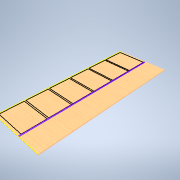
# Autodesk Inventor part: Onderkant1
Saved by Autodesk Inventor 2021 (Build 250183000, 183)
## iProperties
Created: 2021-03-18
Part Number: Onderkant1
Material: Wood (Cherry)
Document SubType Name: Modeling
Designer: ZiweZhang
Density: 0.63 g/cm^3
Appearance: Cherry - Natural Low Gloss
Author: ZiweZhang
Autodesk Inventor part; units mm, degrees
ref_plane "YZ Plane" through (0, 0, 0) normal (1, 0, 0) x (0, 1, 0)
ref_plane "XZ Plane" through (0, 0, 0) normal (0, 1, 0) x (-1, 0, 0)
ref_plane "XY Plane" through (0, 0, 0) normal (0, 0, 1) x (1, 0, 0)
sketch "Sketch1" plane through (0, 0, 0) normal (0, 1, 0) x (-1, 0, 0)
  line L0 (181, 491) -> (-181, 491)
  line L1 (-181, 491) -> (-181, -491)
  line L2 (-181, -491) -> (181, -491)
  line L3 (181, -491) -> (181, 491)
  line L4 (181, 491) -> (-181, -491) construction
  line L5 (-181, 491) -> (181, -491) construction
  point P0 (0, 0)
  dimension "d0" = 362
  dimension "d1" = 982
  constraints: 12 end point, 2 midpoint, 2 parallel, 1 horizontal, 1 perpendicular
  measures "d0" distance of L2.end L1.end
  measures "d1" distance of L1.end L0.end
extrude "Extrusion1" add sketch "Sketch1" along normal blind 6
sketch "Sketch2" plane through (0, 6, 0) normal (0, 1, 0) x (1, 0, 0)
  line L0 (-174, -475) -> (26, -475)
  line L1 (26, -475) -> (26, -325)
  line L2 (26, -325) -> (-174, -325)
  line L3 (-174, -325) -> (-174, -475)
  line L4 (-174, -315) -> (26, -315)
  line L5 (26, -315) -> (26, -165)
  line L6 (26, -165) -> (-174, -165)
  line L7 (-174, -165) -> (-174, -315)
  line L8 (-174, -155) -> (26, -155)
  line L9 (26, -155) -> (26, -5)
  line L10 (26, -5) -> (-174, -5)
  line L11 (-174, -5) -> (-174, -155)
  line L12 (-174, 5) -> (26, 5)
  line L13 (26, 5) -> (26, 155)
  line L14 (26, 155) -> (-174, 155)
  line L15 (-174, 155) -> (-174, 5)
  line L16 (-174, 165) -> (26, 165)
  line L17 (26, 165) -> (26, 315)
  line L18 (26, 315) -> (-174, 315)
  line L19 (-174, 315) -> (-174, 165)
  line L20 (-174, 325) -> (26, 325)
  line L21 (26, 325) -> (26, 475)
  line L22 (26, 475) -> (-174, 475)
  line L23 (-174, 475) -> (-174, 325)
  line L24 (-181, -491) -> (181, -491) projected
  line L25 (-181, 491) -> (-181, -491) projected
  line L26 (27, -489) -> (33, -489)
  line L27 (33, -489) -> (33, 481)
  line L28 (33, 481) -> (27, 481)
  line L29 (27, 481) -> (27, -489)
  point P0 (0, 0)
  dimension "d4" = 200
  dimension "d5" = 150
  dimension "d8" = 160
  dimension "d13" = 16
  dimension "d14" = 7
  dimension "d15" = 6
  dimension "d16" = 970
  constraints: 56 end point, 4 parallel, 2 horizontal, 2 perpendicular, 1 collinear, 1 vertical, 39 other
  measures "d4" distance of L2.end L1.end
  measures "d5" distance of L1.end L0.end
  measures "d8" distance of L0.start L4.start
  measures "d13" distance between parallel lines of L0 L24
  measures "d14" distance between parallel lines of L25 L3
  measures "d15" distance of L28.end L27.end
  measures "d16" distance of L27.end L26.end
body "Solid1"
